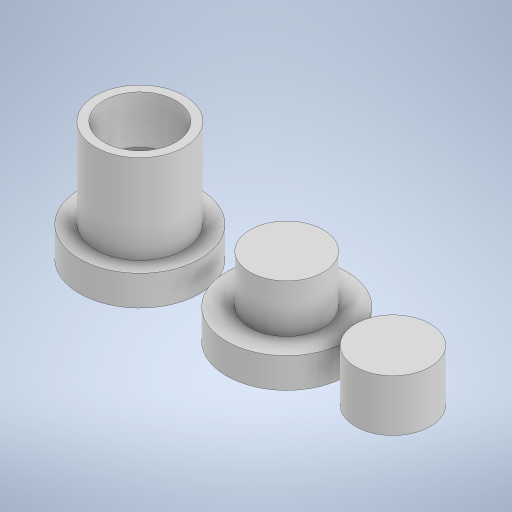
# Autodesk Inventor part: Multiboard Thread insert
Saved by Autodesk Inventor 2024.3 (Build 283343000, 343)
## iProperties
Created: 2024-11-06
Part Number: Multiboard Thread insert
Material: Generic
Document SubType Name: Modeling
Designer: wszaf
Density: 1 g/cm^3
Appearance: Default
Author: wszaf
Autodesk Inventor part; units mm, degrees
ref_plane "YZ Plane" through (0, 0, 0) normal (1, 0, 0) x (0, 1, 0)
ref_plane "XZ Plane" through (0, 0, 0) normal (0, 1, 0) x (-1, 0, 0)
ref_plane "XY Plane" through (0, 0, 0) normal (0, 0, 1) x (1, 0, 0)
sketch "Sketch4" plane through (0, 0, 0) normal (0, 1, 0) x (-1, 0, 0)
  circle A0 centre (0, 0) radius 3.05
  circle A1 centre (0, 0) radius 5
  circle A2 centre (-12.0305, -0.1757) radius 3.05
  circle A3 centre (-12.0305, -0.1757) radius 5
  circle A4 centre (-21.0308, 0) radius 3.1
  dimension "d13" = 6.1
  dimension "d14" = 10
  dimension "d25" = 6.1
  dimension "d26" = 10
  dimension "d30" = 6.2
  constraints: 5 centre point, 4 coincident
  measures "d13" diameter of A0
  measures "d14" diameter of A1
  measures "d25" diameter of A2
  measures "d26" diameter of A3
  measures "d30" diameter of A4
extrude "Extrusion5" add sketch "Sketch4" along normal blind 2.5 contours A0 | A1 | A2 | A3
extrude "Extrusion6" cut sketch "Sketch4" along normal blind 2.1 contours A0 | A2
sketch "Sketch5" plane through (0, 2.5, 0) normal (0, 1, 0) x (1, 0, 0)
  circle A0 centre (0, 0) radius 3.7
  dimension "d19" = 7.4
  constraints: 1 centre point, 1 coincident
  measures "d19" diameter of A0
extrude "Extrusion7" add sketch "Sketch5" along normal blind 7.4
sketch "Sketch6" plane through (0, 9.9, 0) normal (0, 1, 0) x (1, 0, 0)
  circle A0 centre (0, 0) radius 3
  dimension "d22" = 6
  constraints: 1 centre point, 1 coincident
  measures "d22" diameter of A0
extrude "Extrusion8" cut sketch "Sketch6" against normal blind 4
sketch "Sketch7" plane through (12.0305, 2.5, -0.1757) normal (0, 1, 0) x (1, 0, 0)
  circle A0 centre (0, 0) radius 3.05
  circle A1 centre (0, 0) radius 5 projected
  point P0 (-12.0305, -0.1757)
  dimension "d27" = 6.1
  constraints: 1 centre point, 1 concentric
  measures "d27" diameter of A0
extrude "Extrusion9" add sketch "Sketch7" along normal blind 4 contours A0
extrude "Extrusion10" add sketch "Sketch4" along normal blind 4.3 contours A4
sketch "Sketch8" plane through (0, 0, 0) normal (0, 1, 0) x (-1, 0, 0)
  circle A0 centre (0, 0) radius 3.05 projected
  circle A1 centre (0, 0) radius 5 projected
  circle A2 centre (-12.0305, -0.1757) radius 5 projected
split body "Split1" sketch "Sketch8" result two bodies curves A1 first body at (3.1896, 7.4333, 0.2575)
split body "Split2" sketch "Sketch8" result two bodies bodies 3 curves A2 first body at (7.5887, 1.6667, -0.8976)
sketch "Sketch9" plane through (12.0305, 0, -0.1757) normal (0, -1, 0) x (1, 0, 0)
  line L0 (-7.9805, 1.6757) -> (-9.9805, 1.6757)
  line L1 (-9.9805, 1.6757) -> (-9.9805, -1.3243)
  line L2 (-9.9805, -1.3243) -> (-7.9805, -1.3243)
  line L3 (-7.9805, -1.3243) -> (-7.9805, 1.6757)
  circle A0 centre (-12.0305, 0.1757) radius 3.05 projected
  line L4 (4.05, 1.5) -> (2.05, 1.5)
  line L5 (2.05, 1.5) -> (2.05, -1.5)
  line L6 (2.05, -1.5) -> (4.05, -1.5)
  line L7 (4.05, -1.5) -> (4.05, 1.5)
  circle A1 centre (0, 0) radius 3.05 projected
  point P0 (-9.9805, 0.1757)
  point P1 (2.05, 0)
  dimension "d33" = 2
  dimension "d34" = 3
  dimension "d35" = 1
  dimension "d36" = 2
  dimension "d37" = 3
  dimension "d38" = 1
  constraints: 16 end point, 4 parallel, 2 horizontal, 2 horizontal alignment, 2 midpoint, 2 perpendicular
  measures "d33" distance of L2.end L1.end
  measures "d34" distance of L1.end L0.end
  measures "d35" distance edge to line of A0 L1
  measures "d36" distance of L6.end L5.end
  measures "d37" distance of L5.end L5.start
  measures "d38" distance edge to line of A1 L5
extrude "Extrusion11" cut sketch "Sketch9" against normal blind 2.3 contours L3 L2 A0 L0 | A0 L2 L1 L0 | L7 L6 A1 L4 | A1 L6 L5 L4 picked at (-9.6472, 0.1757) picked at (2.3833, 0) bodies 4 2
equation "\"d19\" = Shaft_Diameter - Shaft_Fit_Loose"
equation "\"d20\" = Shaft_Width + Shaft_Width_Free_Space"
equation "\"Shaft_Diameter\" = 8"
equation "\"Shaft_Fit_Loose\" = 0.6"
equation "\"Shaft_Width\" = 7"
equation "\"Shaft_Width_Free_Space\" = 0.4"
